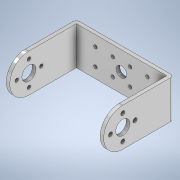
# Autodesk Inventor part: Part2
Saved by Autodesk Inventor 2021 (Build 250183000, 183)
## iProperties
Created: 2021-10-22
Part Number: Part2
Material: Generic
Document SubType Name: Modeling
Designer: Asus
Density: 1 g/cm^3
Appearance: Default
Author: Asus
Autodesk Inventor part; units mm, degrees
ref_plane "YZ Plane" through (0, 0, 0) normal (1, 0, 0) x (0, 1, 0)
ref_plane "XZ Plane" through (0, 0, 0) normal (0, 1, 0) x (-1, 0, 0)
ref_plane "XY Plane" through (0, 0, 0) normal (0, 0, 1) x (1, 0, 0)
sketch "Sketch1" plane through (0, 0, 0) normal (0, 0, 1) x (1, 0, 0)
  line L0 (0, 0) -> (55.6, 0)
  line L1 (55.6, 0) -> (55.6, 21.8)
  line L2 (55.6, 21.8) -> (0, 21.8)
  line L3 (0, 21.8) -> (0, 0)
  dimension "d2" = 21.8
  constraints: 8 end point, 2 parallel, 1 horizontal, 1 perpendicular
  measures "d2" distance of L1.end L0.end
extrude "Extrusion1" add sketch "Sketch1" along normal blind 2
sketch "Sketch2" plane through (0, 0, 2) normal (0, 0, 1) x (1, 0, 0)
  line L0 (0, 21.8) -> (0, 0) projected
  line L1 (55.6, 21.8) -> (0, 21.8) projected
  line L2 (0, 0) -> (2, 0)
  line L3 (2, 0) -> (2, 21.8)
  line L4 (2, 21.8) -> (0, 21.8)
  line L5 (0, 21.8) -> (0, 0)
  line L6 (0, 0) -> (55.6, 0) projected
  line L7 (55.6, 21.8) -> (53.6, 21.8)
  line L8 (53.6, 21.8) -> (53.6, 0)
  line L9 (53.6, 0) -> (55.6, 0)
  line L10 (55.6, 0) -> (55.6, 21.8)
  dimension "d5" = 2
  dimension "d6" = 2
  constraints: 16 end point, 4 parallel, 2 horizontal, 2 perpendicular, 2 point on line
  measures "d5" distance of L4.end L3.end
  measures "d6" distance of L9.end L8.end
extrude "Extrusion2" add sketch "Sketch2" along normal blind 38 contours L1 L3 L2 L0 | L1 L10 L6 L8
fillet "Fillet1" radius 10.9 4 edges at (54.6, 21.8, 40) (54.6, 0, 40) (1, 0, 40) (1, 21.8, 40)
fillet "Fillet2" radius 2 2 edges at (55.6, 10.9, 0) (0, 10.9, 0)
sketch "Sketch3" plane through (55.6, 10.9, 29.1) normal (1, 0, 0) x (0, 0, -1)
  arc A0 (0, 10.9) -> (0, -10.9) centre (0, 0) ccw projected
  circle A1 centre (0, 0) radius 1
  point P0 (29.1, -10.9)
  dimension "d12" = 2
  constraints: 1 centre point, 1 coincident
  measures "d12" diameter of A1
hole "Hole1" at (55.6, 10.9, 29.1) direction (-1, 0, 0) diameter 8 depth 70
sketch "Sketch4" plane through (55.6, 10.9, 29.1) normal (1, 0, 0) x (0, 0, -1)
  circle A0 centre (0, 0) radius 4 projected
  circle A1 centre (0, 0) radius 7
  circle A2 centre (0, 7) radius 1
  circle A3 centre (-7, 0) radius 1
  circle A4 centre (0, -7) radius 1
  circle A5 centre (7, 0) radius 1
  point P0 (29.1, -10.9)
  dimension "d22" = 14
  dimension "d23" = 2
  dimension "d26" = 360
  constraints: 4 centre point, 1 coincident, 1 vertical alignment, 11 other
  measures "d23" diameter of A2
hole "Hole2" at (55.6, 17.9, 29.1) at (55.6, 10.9, 22.1) at (55.6, 3.9, 29.1) at (55.6, 10.9, 36.1) direction (-1, 0, 0) diameter 2 depth 70
thread "Thread2" size "M2x0.4" class "6H" standard "ANSI Metric M Profile" length 4
thread "Thread3" size "M2x0.4" class "6H" standard "ANSI Metric M Profile" length 4
thread "Thread4" size "M2x0.4" class "6H" standard "ANSI Metric M Profile" length 4
thread "Thread5" size "M2x0.4" class "6H" standard "ANSI Metric M Profile" length 4
thread "Thread7" size "M2x0.4" class "6H" standard "ANSI Metric M Profile" length 5
thread "Thread8" size "M2x0.4" class "6H" standard "ANSI Metric M Profile" length 5
thread "Thread9" size "M2x0.4" class "6H" standard "ANSI Metric M Profile" length 5
thread "Thread10" size "M2x0.4" class "6H" standard "ANSI Metric M Profile" length 5
chamfer "Chamfer2" distance 0.2 angle 45 8 edges at (55.6, 10.9, 37.1) (55.6, 3.9, 30.1) (55.6, 10.9, 23.1) (55.6, 17.9, 30.1) (0, 10.9, 37.1) (0, 17.9, 30.1) (0, 3.9, 30.1) (0, 10.9, 23.1)
sketch "Sketch5" plane through (0, 0, 0) normal (0, 0, -1) x (-1, 0, 0)
  line L0 (-53.6, 21.8) -> (-2, 21.8) projected
  line L1 (-27.8, 21.8) -> (-27.8, 0)
  circle A0 centre (-27.8, 10.9) radius 3
  circle A1 centre (-27.8, 10.9) radius 7
  line L2 (-27.8, 10.9) -> (-40.3616, 10.9)
  line L3 (-27.8, 10.9) -> (-34.2529, 17.3529)
  line L4 (-27.8, 10.9) -> (-18.6742, 10.9) construction
  circle A2 centre (-32.7497, 15.8497) radius 1
  circle A3 centre (-32.7497, 5.9503) radius 1
  circle A4 centre (-22.8503, 5.9503) radius 1
  circle A5 centre (-22.8503, 15.8497) radius 1
  line L5 (-32.7497, 15.8497) -> (-42.6487, 15.8497)
  circle A6 centre (-42.6487, 15.8497) radius 1
  circle A7 centre (-42.6487, 5.9503) radius 1
  line L6 (-22.8503, 15.8497) -> (-12.9513, 15.8497)
  circle A8 centre (-12.9513, 15.8497) radius 1
  circle A9 centre (-12.9513, 5.9503) radius 1
  point P0 (0, 0)
  dimension "d60" = 14
  dimension "d59" = 6
  dimension "d61" = 135
  dimension "d62" = 2
  dimension "d65" = 360
  dimension "d67" = 9.899
  dimension "d68" = 2
  dimension "d69" = 2
  dimension "d70" = 9.899
  dimension "d71" = 2
  dimension "d72" = 2
  constraints: 12 end point, 9 centre point, 4 horizontal, 3 coincident, 2 midpoint, 1 equal length, 1 point on line, 1 vertical, 12 other
  measures "d59" diameter of A0
  measures "d61" angle of L4 L3
  measures "d62" diameter of A2
  measures "d67" distance of L5.start L5.end
  measures "d68" diameter of A6
  measures "d69" diameter of A7
  measures "d70" distance of L6.start L6.end
  measures "d71" diameter of A8
  measures "d72" diameter of A9
hole "Hole3" at (42.6487, 15.8497, 0) at (32.7497, 15.8497, 0) at (22.8503, 15.8497, 0) at (12.9513, 15.8497, 0) at (12.9513, 5.9503, 0) at (22.8503, 5.9503, 0) at (32.7497, 5.9503, 0) at (42.6487, 5.9503, 0) direction (0, 0, 1) diameter 2 depth 3
sketch "Sketch6" plane through (0, 0, 0) normal (0, 0, -1) x (-1, 0, 0)
  line L0 (-2, 0) -> (-53.6, 0) projected
  line L1 (-27.8, 0) -> (-27.8, 21.8)
  line L2 (-53.6, 21.8) -> (-2, 21.8) projected
  circle A0 centre (-27.8, 10.9) radius 3
  point P0 (0, 0)
  dimension "d80" = 6
  constraints: 3 midpoint, 2 end point, 1 centre point
  measures "d80" diameter of A0
hole "Hole4" at (27.8, 10.9, 0) direction (0, 0, 1) diameter 6 depth 3
chamfer "Chamfer3" distance 0.2 angle 45 8 edges at (12.9513, 4.9503, 0) (22.8503, 4.9503, 0) (32.7497, 4.9503, 0) (42.6487, 4.9503, 0) (12.9513, 14.8497, 0) (22.8503, 14.8497, 0) (32.7497, 14.8497, 0) (42.6487, 14.8497, 0)
body "Solid1"
